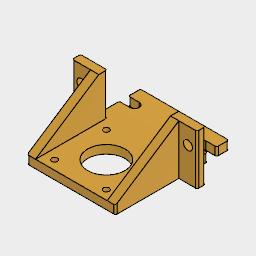
Z_Motor_Mount_1.0_F01 (Autodesk Fusion 360 design; units mm, degrees)
Autodesk Fusion 360 part; units mm, degrees
sketch "スケッチ1" plane through (0, 0, 0) normal (0, 0, 1) x (1, 0, 0)
  line L0 (-26.5, 47) -> (26.5, 47)
  line L1 (26.5, 47) -> (26.5, -21)
  line L2 (26.5, -21) -> (-26.5, -21)
  line L3 (-26.5, -21) -> (-26.5, 47)
  circle A0 centre (0, 0) radius 11.2
  circle A1 centre (-15.5, -15.5) radius 1.75
  circle A2 centre (15.5, -15.5) radius 1.75
  circle A3 centre (15.5, 15.5) radius 1.75
  circle A4 centre (-15.5, 15.5) radius 1.75
  line L4 (21.5, 17) -> (37.5, 17)
  line L5 (37.5, 17) -> (37.5, 22)
  line L6 (37.5, 22) -> (21.5, 22)
  line L7 (21.5, 22) -> (21.5, 17)
  circle A5 centre (20, 37) radius 2.7
  line L8 (0, 0) -> (0, 47) construction
  line L9 (-37.5, 22) -> (-21.5, 22)
  line L10 (-21.5, 22) -> (-21.5, 17)
  line L11 (-21.5, 17) -> (-37.5, 17)
  line L12 (-37.5, 17) -> (-37.5, 22)
  circle A6 centre (-20, 37) radius 2.7
  line L13 (26.5, 39.7) -> (20, 39.7)
  line L14 (26.5, 34.3) -> (20, 34.3)
  line L15 (-26.5, 34.3) -> (-20, 34.3)
  line L16 (-26.5, 39.7) -> (-20, 39.7)
  dimension "d1" = 53
  dimension "d2" = 68
  dimension "d3" = 26.5
  dimension "d4" = 21
  dimension "d5" = 22.4
  dimension "d6" = 3.5
  dimension "d7" = 15.5
  dimension "d8" = 15.5
  dimension "d10" = 360
  dimension "d11" = 16
  dimension "d12" = 5
  dimension "d13" = 11
  dimension "d14" = 25
  dimension "d15" = 5.4
  dimension "d16" = 10
  dimension "d17" = 6.5
  measures "d1" distance of L1 L3
  measures "d2" distance of L0 L2
  measures "d3" distance of A0.centre L1
  measures "d4" distance of A0.centre L2
  measures "d5" diameter of A0
  measures "d6" diameter of A1
  measures "d7" distance of A0.centre A1.centre
  measures "d8" distance of A0.centre A1.centre
  measures "d11" distance of L4.start L4.end
  measures "d12" distance of L4.start L6.end
  measures "d13" distance of L1 L5
  measures "d14" distance of L0 L6
  measures "d15" diameter of A5
  measures "d16" distance of L0 A5.centre
  measures "d17" distance of L1 A5.centre
extrude "押し出し1" add sketch "スケッチ1" along normal blind 5 contours L0 L1 L2 L3 L4 L6 L7 A5 L9 L10 L11 A6 L13 L14 L15 L16
extrude "押し出し2" add sketch "スケッチ1" along normal blind 30 contours L3 L9 L10 L11 | L3 L9 L11 L12 | L1 L4 L5 L6 | L1 L4 L6 L7
chamfer "面取り1" distance 38 distance2 25 2 edges at (24, 17, 5) (-24, 17, 5) measured on face at (0.279, 27.7319, 5) measured on face at (0.279, 27.7319, 5)
fillet "フィレット1" radius 1 14 edges at (-37.5, 17, 15) (-37.5, 22, 15) (-26.5, -21, 2.5) (-26.5, 34.3, 2.5) (-26.5, 39.7, 2.5) (-26.5, 47, 2.5) (26.5, 47, 2.5) (26.5, 39.7, 2.5) (26.5, 34.3, 2.5) (37.5, 22, 15) (37.5, 17, 15) (21.5, 22, 17.5) (-21.5, 22, 17.5) (26.5, -21, 2.5)
hole "穴1" at (-32, 17, 20) direction (0, 1, 0) diameter 5.4 depth 11 tip angle 118
mirror "ミラー1" about plane through (0, 0, 0) normal (1, 0, 0) of "穴1"
equation "d3 = d1 / 2"
